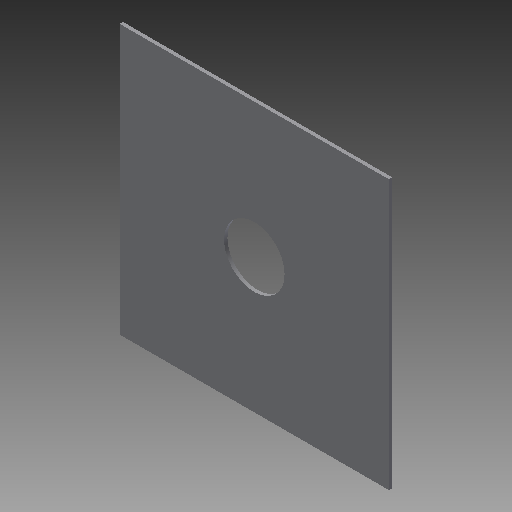
# Autodesk Inventor part: mountingPanelCannon
Saved by Autodesk Inventor 2017 (Build 210142000, 142)
## iProperties
Created: 2016-04-20
Part Number: mountingPanelCannon
Material: Generic
Document SubType Name: Modeling
Designer: Administrator
Density: 1 g/cm^3
Appearance: Default
Author: Administrator
Autodesk Inventor part; units mm, degrees
ref_plane "YZ Plane" through (0, 0, 0) normal (1, 0, 0) x (0, 1, 0)
ref_plane "XZ Plane" through (0, 0, 0) normal (0, 1, 0) x (-1, 0, 0)
ref_plane "XY Plane" through (0, 0, 0) normal (0, 0, 1) x (1, 0, 0)
sketch "Sketch1" plane through (0, 0, 0) normal (0, 0, 1) x (1, 0, 0)
  line L0 (25.4, 63.5) -> (-101.6, 63.5)
  line L1 (-101.6, 63.5) -> (-101.6, 190.5)
  line L2 (-101.6, 190.5) -> (25.4, 190.5)
  line L3 (25.4, 190.5) -> (25.4, 63.5)
  point P0 (0, 0)
  dimension "d0" = 127
  dimension "d1" = 127
  constraints: 8 end point, 2 parallel, 1 horizontal, 1 perpendicular
  measures "d0" distance of L1.end L2.end
  measures "d1" distance of L0.end L1.end
extrude "Extrusion1" add sketch "Sketch1" along normal blind 1.5875
sketch "Sketch2" plane through (0, 0, 0) normal (0, 0, -1) x (-1, 0, 0)
  line L0 (-25.4, 63.5) -> (101.6, 63.5) projected
  line L1 (101.6, 63.5) -> (101.6, 190.5) projected
  line L2 (101.6, 190.5) -> (-25.4, 190.5) projected
  line L3 (-25.4, 190.5) -> (-25.4, 63.5) projected
  line L4 (38.1, 190.5) -> (38.1, 127)
  point P0 (0, 0)
  dimension "d4" = 127
  dimension "d5" = 127
  dimension "d6" = 63.5
  constraints: 2 end point, 1 coincident, 1 midpoint, 1 parallel
  measures "d4" distance between parallel lines of L0 L2
  measures "d5" distance between parallel lines of L1 L3
  measures "d6" distance of L4.start L4.end
hole "Hole1" at (-38.1, 127, 0) direction (0, 0, 1) diameter 28.575 end through all
body "Solid1"
